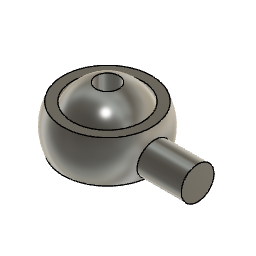
deltaFusionFile (Autodesk Fusion 360 archive; units mm, degrees)
design "rod end bearing"
Autodesk Fusion 360 part; units mm, degrees
sketch "Sketch1" plane through (0, 0, 0) normal (0, 1, 0) x (1, 0, 0)
  circle A0 centre (0, 0) radius 6
  circle A1 centre (0, 0) radius 6.25
  circle A2 centre (0, 0) radius 7.5
  line L0 (0, 7.5) -> (0, -7.5)
  line L1 (0, -1.75) -> (0, -22.5)
  line L2 (0, 0) -> (17, 0) construction
  line L3 (-6.7831, -3.2) -> (6.7831, -3.2)
  line L4 (-6.7831, 3.2) -> (6.7831, 3.2)
  line L5 (-1.75, -5.7391) -> (-1.75, 5.7391)
  line L6 (1.75, -5.7391) -> (1.75, 5.7391)
  line L7 (6.7831, 3.2) -> (13.7831, 3.2)
  line L8 (13.7831, 3.2) -> (13.7831, -1.8)
  line L9 (13.7831, -1.8) -> (6.7831, -1.8)
  line L10 (6.7831, -1.8) -> (6.7831, 3.2)
  line L11 (6.7831, 0.7) -> (13.7831, 0.7)
  dimension "d2" = 12
  dimension "d3" = 12.5
  dimension "d5" = 15
  dimension "d7" = 3.2
  dimension "d9" = 3.2
  dimension "d11" = 1.75
  dimension "d12" = 1.75
  dimension "d14" = 5
  dimension "d15" = 7
  constraint coincident A0.centre A1.centre
  constraint concentric A0 A1
  constraint coincident A2 L0.start
  constraint coincident A2 L0.end
  constraint vertical L0
  constraint collinear L0 L1
  constraint perpendicular L0 L2
  constraint coincident A2 L3.start
  constraint coincident A2 L3.end
  constraint horizontal L3
  constraint coincident A2 L4.start
  constraint coincident A2 L4.end
  constraint perpendicular L0 L4
  constraint coincident A0 L5.start
  constraint coincident A0 L5.end
  constraint perpendicular L3 L5
  constraint coincident A0 L6.start
  constraint coincident A0 L6.end
  constraint perpendicular L4 L6
  constraint horizontal L7
  constraint vertical L8
  constraint horizontal L9
  constraint vertical L10
  constraint midpoint L10 L11.start
  constraint midpoint L8 L11.end
  measures "d2" diameter of A0
  measures "d3" diameter of A1
  measures "d5" diameter of A2
  measures "d7" distance of L2 L3
  measures "d9" distance of L2 L4
  measures "d11" distance of L0 L5
  measures "d12" distance of L0 L6
  measures "d14" distance of L4.end L9.end
  measures "d15" distance of L8 L10
revolve "Revolve1" add sketch "Sketch1" angle 360 about axis through (0, 0, -7.5) along (0, 0, 1) contours A0 L3 L4 L6 | A0 L3 L6 | A1 A2 L3 L4 L9 L10 | A2 L10 L11 | A2 L9 L10 L11 makes body 1 at (5.1953, -2.9995, -0.1088) makes body 2 at (-3.7484, -6.4924, -0.2204)
revolve "Revolve2" add sketch "Sketch1" angle 360 about axis through (6.7831, 0, -0.7) along (1, 0, 0) contours A2 L8 L9 L11 | A2 L9 L10 L11 bodies 2
equation "ballDia = 12 mm"
equation "d2 = ballDia"
equation "d3 = ballDia + spacing * 2"
equation "outerDia = 15 mm"
equation "d5 = outerDia"
equation "spacing = 0.25 mm"
equation "d7 = ballHeight"
equation "ballHeight = 3.2 mm"
equation "d9 = ballHeight"
equation "innerShaftDia = 3.5 mm"
equation "d11 = innerShaftDia / 2"
equation "d12 = innerShaftDia / 2"
equation "d15 = connectorLen"
equation "connectorLen = 7 mm"

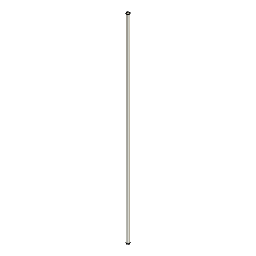
design "200mm alu rod"
Autodesk Fusion 360 part; units mm, degrees
sketch "Sketch1" plane through (0, 0, 0) normal (0, 0, 1) x (1, 0, 0)
  circle A0 centre (0, 0) radius 1.5
  dimension "d1" = 3
  constraint coincident A0.centre origin
  measures "d1" diameter of A0
extrude "Extrude1" add sketch "Sketch1" along normal blind 200

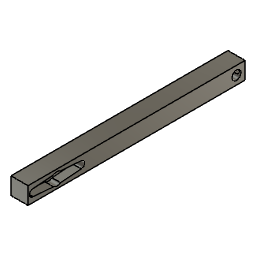
design "forearm"
Autodesk Fusion 360 part; units mm, degrees
sketch "Sketch1" plane through (0, 0, 0) normal (1, 0, 0) x (0, 1, 0)
  line L0 (-15.7621, -1.2) -> (15.7621, -1.2)
  arc A0 (-14.1, 2.05) -> (-14.1, -2.05) centre (-14.1, 0) ccw
  line L1 (14.1, 2.05) -> (2.0791, 3)
  line L2 (-14.1, -2.05) -> (-2.0791, -3)
  arc A1 (14.1, -2.05) -> (14.1, 2.05) centre (14.1, 0) ccw
  line L3 (-2.0791, -3) -> (-14.1, -2.05)
  line L4 (-2.0791, 3) -> (-14.1, 2.05)
  line L5 (2.0791, -3) -> (14.1, -2.05)
  circle A2 centre (0, 0) radius 2.3
  circle A3 centre (0, 0) radius 2.3
  line L6 (2.0791, 3) -> (14.1, 2.05)
  line L7 (-2.0791, 3) -> (2.0791, 3) construction
  line L8 (2.0791, -3) -> (14.1, -2.05)
  line L9 (-2.0791, 3) -> (-14.1, 2.05)
  line L10 (-2.0791, -3) -> (2.0791, -3) construction
  circle A4 centre (0, 0) radius 3.65
  line L11 (-15.7621, 1.2) -> (15.7621, 1.2)
  line L12 (-14.1, 0) -> (14.1, 0) construction
  line L13 (1.75, 0) -> (22.5, 0) construction
  line L14 (-14.1, 2.05) -> (-14.1, -2.05) construction
  line L15 (14.1, 2.05) -> (14.1, -2.05) construction
  line L16 (-17, -5) -> (110, -5)
  line L17 (110, -5) -> (110, 5)
  line L18 (110, 5) -> (-17, 5)
  line L19 (-17, 5) -> (-17, -5)
  circle A5 centre (105, 0) radius 2.625
  point P0 (-12.2301, 0)
  point P1 (-12.2301, 0)
  dimension "d1" = 4.6
  dimension "d2" = 2.05
  dimension "d3" = 14.1
  dimension "d4" = 7.3
  dimension "d5" = 2.05
  dimension "d6" = 14.1
  dimension "d7" = 3
  dimension "d8" = 3
  dimension "d9" = 1.2
  dimension "d10" = 1.2
  dimension "d11" = 127
  dimension "d12" = 10
  dimension "d13" = 5
  dimension "d14" = 17
  dimension "d26" = 5.25
  dimension "d40" = 5
  constraint coincident P1 P0
  constraint coincident L2.end A4
  constraint coincident L1.start A1.end
  constraint coincident A1.start L5.end
  constraint coincident L2.end L3.start
  constraint coincident A0.start L4.end
  constraint coincident L0.start A0
  constraint horizontal L0
  constraint coincident L11.end A1
  constraint parallel L0 L11
  constraint coincident A2.centre A3.centre
  constraint coincident L5.start A4
  constraint horizontal L10
  constraint coincident L1.end A4
  constraint parallel L7 L11
  constraint coincident L0.end A1
  constraint coincident L11.start A0
  constraint coincident L4.start A4
  constraint coincident A0.centre L12.start
  constraint coincident A1.centre L12.end
  constraint collinear L12 L13
  constraint coincident A0.centre L14
  constraint coincident A1.centre L15
  constraint perpendicular L12 L15
  constraint perpendicular L12 L14
  constraint horizontal L16
  constraint vertical L17
  constraint horizontal L18
  constraint vertical L19
  measures "d1" diameter of A2
  measures "d2" radius of A0
  measures "d3" distance of A2.centre A0.centre
  measures "d4" diameter of A4
  measures "d5" radius of A1
  measures "d6" distance of A2.centre A1.centre
  measures "d7" distance of A2.centre L10
  measures "d8" distance of A2.centre L7
  measures "d9" distance of L11 L12
  measures "d10" distance of L0 L12
  measures "d11" distance of L16.start L16.end
  measures "d12" distance of L16.start L18.end
  measures "d13" distance of A2.centre L18
  measures "d14" distance of A2.centre L19
  measures "d26" diameter of A5
  measures "d40" distance of L17 A5.centre
extrude "Extrude1" add sketch "Sketch1" along normal blind 10
extrude "Extrude2" add sketch "Sketch1" along normal blind 5 contours L0 A0 L2 L3 A4 | L0 A2 A3 A4 | A0 L4 L9 A4 L11 | A2 A3 A4 L11 | L0 A1 L5 L8 A4 | L1 A1 L6 A4 L11
extrude "Extrude3" cut sketch "Sketch1" along normal blind 2.5 contours L0 A0 L2 L3 A4 | L0 A2 A3 A4 | A0 L4 L9 A4 L11 | A2 A3 A4 L11 | L0 A1 L5 L8 A4 | L1 A1 L6 A4 L11
sketch "Sketch2" plane through (0, 110, 0) normal (0, 1, 0) x (-1, 0, 0)
  line L0 (0, -5) -> (0, 5)
  line L1 (0, 5) -> (-10, 5)
  line L2 (-10, 5) -> (-10, -5)
  line L3 (-10, -5) -> (0, -5)
  line L4 (0, 0) -> (-10, 0) construction
  circle A0 centre (-2.5, 0) radius 1.5
  circle A1 centre (-7.5, 0) radius 1.5
  dimension "d27" = 3
  dimension "d28" = 3
  dimension "d29" = 2.5
  dimension "d30" = 2.5
  constraint coincident L4.start origin
  constraint midpoint L2 L4.end
  constraint coincident L4 A0.centre
  constraint coincident L4 A1.centre
  measures "d27" diameter of A0
  measures "d28" diameter of A1
  measures "d29" distance of L2 A1.centre
  measures "d30" distance of L0 A0.centre
extrude "Extrude4" cut sketch "Sketch2" against normal blind 5 contours A0 | A1
extrude "Extrude5" add sketch "Sketch1" along normal blind 5.5 contours A5
extrude "Extrude6" cut sketch "Sketch1" along normal blind 4.5 contours A5
ref_plane "WorkPlane1" through (5, 100, 0) normal (0, -1, 0) x (0, 0, -1)
split "Split1" [suppressed]
equation "d11 = 100 mm + 17 mm + 10 mm"
